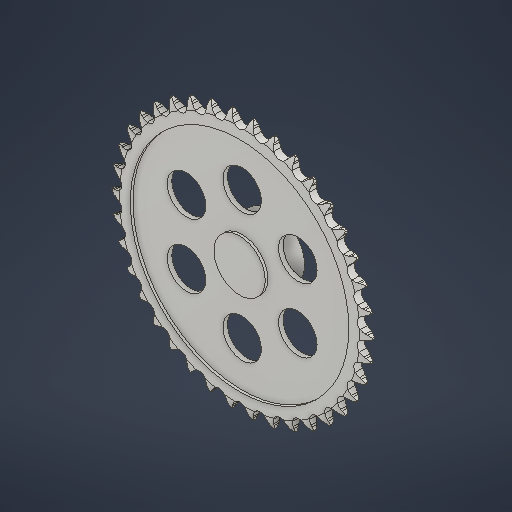
# Autodesk Inventor part: Roller Chain Sprocket1
Saved by Autodesk Inventor 2026.1 (Build 301233020, 233B)
## iProperties
CustomPartVersion: 1
Created: 2025-12-30
Part Number: Roller Chain Sprocket1
Material: Steel
Document SubType Name: Modeling
Designer: Austin Ngobeni
Density: 1 g/cm^3
Appearance: Steel
Author: Austin Ngobeni
Autodesk Inventor part; units mm, degrees
ref_plane "YZ Plane" through (0, 0, 0) normal (1, 0, 0) x (0, 1, 0)
ref_plane "XZ Plane" through (0, 0, 0) normal (0, 1, 0) x (-1, 0, 0)
ref_plane "XY Plane" through (0, 0, 0) normal (0, 0, 1) x (1, 0, 0)
sketch "Theoretical Tooth Profile" plane through (0, 0, 0) normal (0, 0, 1) x (1, 0, 0)
  circle A0 centre (0, 0) radius 48.4383 construction
  line L0 (0, 0) -> (0, 48.4383) construction
  line L1 (0, 0) -> (7.9727, 47.7776) construction
  circle A1 centre (0, 0) radius 50.6728
  arc A2 (-2.0277, 46.9335) -> (2.0277, 46.9335) centre (0, 48.4383) ccw
  line L2 (0, 48.4383) -> (7.9727, 47.7776) construction
  line L3 (0, 48.4383) -> (3.2121, 50.822) construction
  line L4 (3.2121, 50.822) -> (-2.9173, 48.5847) construction
  arc A3 (3.9087, 50.5218) -> (3.1611, 49.2527) centre (6.9761, 47.8602) ccw
  arc A4 (-3.1611, 49.2527) -> (-3.9087, 50.5218) centre (-6.9761, 47.8602) ccw
  line L5 (-6.9761, 47.8602) -> (-3.1611, 49.2527) construction
  arc A5 (-2.9173, 48.5847) -> (-2.0277, 46.9335) centre (3.2121, 50.822) ccw
  line L6 (-2.9173, 48.5847) -> (-3.1611, 49.2527)
  arc A6 (2.0277, 46.9335) -> (2.9173, 48.5847) centre (-3.2121, 50.822) ccw
  line L7 (3.1611, 49.2527) -> (2.9173, 48.5847)
  line L8 (0, 0) -> (4.1845, 50.4997) construction
  point P0 (3.9863, 48.1079)
  dimension "d0" = 96.8765
  dimension "d2" = 9.474
  dimension "d3" = 2.525
  dimension "d10" = 126.579
  dimension "d11" = 16.526
  dimension "d12" = 4
  dimension "d13" = 6.525
  dimension "d14" = 7
  dimension "d23" = 2.4
  constraints: 18 end point, 15 point on circle, 7 centre point, 3 coincident, 3 point on line, 3 symmetric about line, 3 tangent, 1 equal radius, 1 midpoint, 1 parallel, 1 vertical, 1 other
  measures "d0" diameter of A0
  measures "d2" angle of L1 L0
  measures "d3" radius of A2
  measures "d10" angle of L3 L0
  measures "d11" angle of L4 L3
  measures "d12" distance of L2.start L3.end
  measures "d13" distance of L3.end L4.end
  measures "d14" distance of A3.centre L0.end
  measures "d23" distance from line of L8.end L2
sketch "Tooth Profile" plane through (0, 0, 0) normal (0, 0, 1) x (1, 0, 0)
  arc A0 (-2.3544, 47.5258) -> (2.3544, 47.5258) centre (0, 48.4383) ccw
  arc A1 (3.7662, 50.5327) -> (2.3544, 47.5258) centre (24.7325, 38.853) ccw
  arc A2 (-2.3544, 47.5258) -> (-3.7662, 50.5327) centre (-24.7325, 38.853) ccw
  line L0 (0, 0) -> (0, 48.4383) construction
  line L1 (0, 48.4383) -> (2.3544, 47.5258) construction
  line L2 (0, 48.4383) -> (-2.3544, 47.5258) construction
  circle A3 centre (0, 0) radius 50.6728 projected
  dimension "d44" = 137.632
  dimension "d45" = 24
  dimension "d46" = 2.525
  constraints: 9 point on circle, 6 end point, 3 centre point, 2 tangent, 1 coincident, 1 equal radius, 1 vertical, 1 other
  measures "d44" angle of L2 L1
  measures "d45" radius of A1
  measures "d46" radius of A0
sketch "Section Profile" plane through (0, 0, 0) normal (1, 0, 0) x (0, 1, 0)
  line L0 (50.6728, 0) -> (-50.6728, 0) projected
  line L1 (40.4556, 1.395) -> (-40.4556, 1.395)
  line L2 (-40.4556, 1.395) -> (-40.4556, -1.395)
  line L3 (-40.4556, -1.395) -> (40.4556, -1.395)
  line L4 (40.4556, -1.395) -> (40.4556, 1.395)
  line L5 (40.4556, 1.395) -> (50.6728, 1.395) construction
  line L6 (50.6728, 1.395) -> (50.6728, -1.395) construction
  line L7 (50.6728, -1.395) -> (40.4556, -1.395) construction
  line L8 (40.4556, -1.395) -> (40.4556, 1.395)
  arc A0 (50.6728, 0.355) -> (46.7284, 1.395) centre (46.7284, -6.605) ccw
  arc A1 (46.7284, -1.395) -> (50.6728, -0.355) centre (46.7284, 6.605) ccw
  line L9 (46.7284, 1.395) -> (0, 1.395)
  line L10 (0, 1.395) -> (0, -1.395)
  line L11 (0, -1.395) -> (46.7284, -1.395)
  line L12 (0, 1.395) -> (0, -1.395)
  line L13 (50.6728, 0.355) -> (50.6728, -0.355)
  point P0 (0, 0)
  point P1 (0, 0)
  dimension "d30" = 2.79
  dimension "d31" = 80.9112
  dimension "d32" = 2.79
  dimension "d33" = 1.04
  dimension "d34" = 8
  dimension "d43" = 1.395
  constraints: 26 end point, 7 midpoint, 5 perpendicular, 4 parallel, 4 point on circle, 3 point on line, 3 symmetric about line, 2 centre point, 2 horizontal, 2 tangent, 1 collinear, 1 other
  measures "d30" distance between parallel lines of L7 L5
  measures "d31" distance between parallel lines of L2 L4
  measures "d32" distance between parallel lines of L3 L1
  measures "d33" distance from line of L13.start L5
  measures "d34" radius of A0
  measures "d43" distance between parallel lines of L3 L0
revolve "Shroud" add sketch "Section Profile" angle 360 about axis through (0, 0, 1.395) along (0, 0, -1) contours L10 L3 L2 L0 | L0 L2 L1 L10
revolve "Strand" add sketch "Section Profile" angle 360 about axis through (0, 0, 1.395) along (0, 0, -1) contours L13 A1 L11 L4 L0 | L0 L4 L9 A0 L13 | L4 L3 L10 L0 | L0 L10 L1 L4
fillet "Fillet2" [suppressed]
pattern_of_one "Strand Pattern"
extrude "Theoretical Tooth" cut sketch "Theoretical Tooth Profile" along normal through all both and the other way through all contours A3 L7 A6 A2 A5 L6 A4 A1 picked at (0.4347, 48.1743)
extrude "Tooth" [suppressed]
pattern_circular "Tooth Pattern" count 38 over 360 about axis through (0, 0, -10) along (0, 0, 1) of "Theoretical Tooth"
ref_plane "Timing Plane" through (0, 48.4383, 0) normal (1, 0, 0) x (0, 1, 0)
sketch "Sketch4" plane through (0, 48.4383, 1.395) normal (0, 0, 1) x (1, 0, 0)
  circle A0 centre (0, -48.4383) radius 42.5
  circle A1 centre (0, -48.4383) radius 10
  circle A2 centre (0, -48.4383) radius 25 construction
  circle A3 centre (0, -23.4383) radius 7.5
  circle A4 centre (-21.6506, -35.9383) radius 7.5
  circle A5 centre (-21.6506, -60.9383) radius 7.5
  circle A6 centre (0, -73.4383) radius 7.5
  circle A7 centre (21.6506, -60.9383) radius 7.5
  circle A8 centre (21.6506, -35.9383) radius 7.5
  dimension "d55" = 50
  dimension "d53" = 85
  dimension "d54" = 20
  dimension "d56" = 15
  dimension "d59" = 360
  constraints: 8 centre point, 3 coincident, 1 vertical alignment, 15 other
  measures "d53" diameter of A0
  measures "d54" diameter of A1
  measures "d56" diameter of A3
extrude "Extrusion4" cut sketch "Sketch4" against normal blind 1
extrude "Extrusion5" cut sketch "Sketch4" against normal through all contours A3 | A4 | A5 | A6 | A7 | A8
sketch "Sketch5" plane through (0, 48.4383, -1.395) normal (0, 0, -1) x (-1, 0, 0)
  circle A0 centre (0, -48.4383) radius 12.5
  circle A1 centre (0, -48.4383) radius 7.5
  dimension "d65" = 25
  dimension "d66" = 5
  constraints: 2 centre point, 1 coincident
  measures "d65" diameter of A0
  measures "d66" radial gap between concentric circles of A0 A1
extrude "Extrusion6" add sketch "Sketch5" along normal blind 10
equation "\"d3\" = 0.5 * da_Dr + da_SC"
equation "\"d12\" = 0.8 * da_Dr"
equation "\"d13\" = 1.3 * da_Dr + da_SC"
equation "\"d14\" = 1.4 * da_Dr"
equation "\"d23\" = da_Ha"
equation "\"d44\" = da_Alfa"
equation "\"d45\" = da_Re"
equation "\"d46\" = da_Ri"
equation "\"d30\" = da_Bf"
equation "\"d31\" = da_Ds"
equation "\"d32\" = da_Bs"
equation "\"d33\" = da_Ba"
equation "\"d34\" = da_Rx"
equation "\"d51\" = da_Ra"
equation "\"d40\" = da_pt"
equation "\"form_type\" = 0"
equation "\"da_p\" = 8"
equation "\"da_Dr\" = 5"
equation "\"da_SC\" = 0.025"
equation "\"da_Ha\" = 2.4"
equation "\"da_pt\" = 5.64"
equation "\"da_Bf\" = 2.79"
equation "\"da_Ba\" = 1.04"
equation "\"da_Rx\" = 8"
equation "\"da_Ra\" = 0.32"
equation "\"da_Bs\" = 2.79"
equation "\"da_Ds\" = 80.91124"
equation "\"da_Re\" = 24"
equation "\"da_Ri\" = 2.525"
equation "\"da_Alfa\" = 137.632deg"
body "Solid1"
